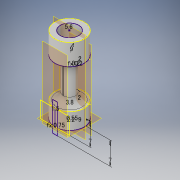
# Autodesk Inventor part: モータジョイント
Saved by Autodesk Inventor 2019.3 (Build 233278000, 278)
## iProperties
Created: 2019-08-08
Part Number: モータジョイント
Material: Generic
Document SubType Name: Modeling
Designer: ushiyama
Density: 1 g/cm^3
Appearance: Default
Author: ushiyama
Autodesk Inventor part; units mm, degrees
ref_plane "YZ Plane" through (0, 0, 0) normal (1, 0, 0) x (0, 1, 0)
sketch "スケッチ2" plane through (0, 0, 0) normal (0, 1, 0) x (-1, 0, 0)
  circle A0 centre (0, 0) radius 4.5
  dimension "d9" = 9
  constraints: 1 centre point, 1 coincident
  measures "d9" diameter of A0
sketch "スケッチ1" plane through (0, 0, 0) normal (0, 1, 0) x (-1, 0, 0)
  arc A0 (-0.55, -0.9526) -> (-0.55, 0.9526) centre (0, 0) ccw
  line L0 (-0.55, -0.9526) -> (-0.55, 0.9526)
  dimension "d0" = 2.2
  dimension "d2" = 0.55
  constraints: 2 end point, 2 point on circle, 1 centre point, 1 coincident, 1 vertical
  measures "d0" diameter of A0
  measures "d2" distance from line of point (0, 0) L0
extrude "押し出し1" add sketch "スケッチ2" along normal blind 5
extrude "押し出し2" cut sketch "スケッチ1" along normal blind 3
ref_plane "作業平面2" through (0, 0, 4.5) normal (0, 0, 1) x (1, 0, 0)
sketch "スケッチ4" plane through (0, 0, 4.5) normal (0, 0, 1) x (1, 0, 0)
  line L0 (4.5, 5) -> (-4.5, 5) projected
  line L1 (-4.5, 0) -> (4.5, 0) projected
  line L2 (4.5, 0) -> (4.5, 5) projected
  line L3 (-4.5, 0) -> (-4.5, 5) projected
  line L4 (-0.75, 7) -> (0.75, 7)
  line L5 (0.75, 7) -> (0.75, -2)
  line L6 (0.75, -2) -> (-0.75, -2)
  line L7 (-0.75, -2) -> (-0.75, 7)
  line L8 (0, 5) -> (0, 0)
  dimension "d14" = 7
  dimension "d15" = 7
  dimension "d16" = 1.5
  dimension "d18" = 0.75
  constraints: 10 end point, 2 parallel, 1 horizontal, 1 midpoint, 1 perpendicular, 1 vertical
  measures "d14" distance between parallel lines of L1 L4
  measures "d15" distance between parallel lines of L0 L6
  measures "d16" distance between parallel lines of L5 L7
  measures "d18" distance between parallel lines of L5 L8
sketch "スケッチ3" plane through (0, 5, 0) normal (0, 1, 0) x (1, 0, 0)
  circle A0 centre (0, 0) radius 4.5 projected
  circle A1 centre (0, 0) radius 1.9
  dimension "d11" = 3.8
  constraints: 1 centre point, 1 coincident
  measures "d11" diameter of A1
extrude "押し出し6" add sketch "スケッチ3" along normal blind 12 contours A1
ref_plane "作業平面3" through (0, 17, 0) normal (0, 1, 0) x (1, 0, 0)
sketch "スケッチ5" plane through (0, 17, 0) normal (0, 1, 0) x (1, 0, 0)
  circle A0 centre (0, 0) radius 4.5 projected
  circle A1 centre (0, 0) radius 4.5
  dimension "d29" = 9
  constraints: 1 centre point, 1 coincident
  measures "d29" diameter of A1
extrude "押し出し8" add sketch "スケッチ5" along normal blind 6.5
sketch "スケッチ7" plane through (0, 23.5, 0) normal (0, 1, 0) x (1, 0, 0)
  circle A0 centre (0, 0) radius 2.8
  circle A1 centre (0, 0) radius 4.5 projected
  dimension "d32" = 5.6
  constraints: 1 centre point, 1 coincident
  measures "d32" diameter of A0
extrude "押し出し9" cut sketch "スケッチ7" against normal blind 4 contours A0
ref_plane "作業平面4" through (0, 5, -1.9) normal (0, 0, 1) x (1, 0, 0)
sketch "スケッチ8" plane through (0, 5, -1.9) normal (0, 0, 1) x (1, 0, 0)
  line L0 (0.2, 10) -> (-0.2, 10)
  line L1 (-0.2, 10) -> (-0.2, 2)
  line L2 (-0.2, 2) -> (0.2, 2)
  line L3 (0.2, 2) -> (0.2, 10)
  line L4 (-4.5, 12) -> (4.5, 12) projected
  line L5 (4.5, 0) -> (-4.5, 0) projected
  line L6 (0, 9.0505) -> (0, 8.9347)
  point P0 (0, -5)
  point P1 (0, 10)
  dimension "d41" = 2
  dimension "d42" = 2
  dimension "d43" = 0.2
  dimension "d44" = 0.2
  constraints: 10 end point, 2 parallel, 2 vertical, 1 horizontal, 1 midpoint, 1 perpendicular
  measures "d41" distance between parallel lines of L4 L0
  measures "d42" distance between parallel lines of L5 L2
  measures "d43" distance between parallel lines of L6 L1
  measures "d44" distance between parallel lines of L6 L3
extrude "押し出し10" cut sketch "スケッチ8" along normal blind 5
fillet "フィレット3" radius 2 2 edges at (-1.9, 5, 0) (-1.9, 17, 0)
equation "\"d18\" = 0.5 * d16"
equation "\"d43\" = d44"
